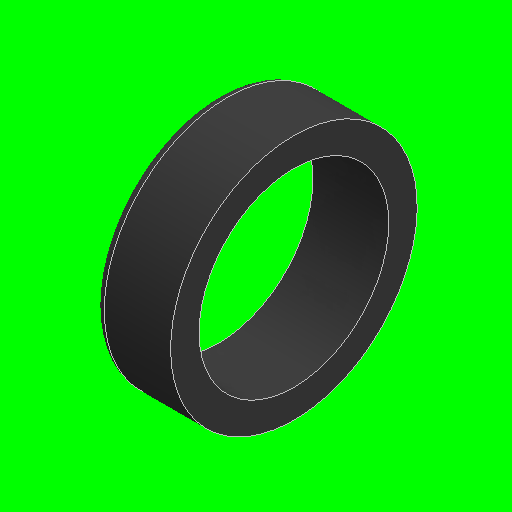
# Autodesk Inventor part: Tire
Saved by Autodesk Inventor 2023 (Build 270158000, 158)
## iProperties
Created: 2022-03-28
Part Number: Tire
Material: ゴム
Document SubType Name: Modeling
Designer: neko2
Density: 0.93 g/cm^3
Appearance: ゴム - 黒
Author: neko2
Autodesk Inventor part; units mm, degrees
ref_plane "YZ Plane" through (0, 0, 0) normal (1, 0, 0) x (0, 1, 0)
ref_plane "XZ Plane" through (0, 0, 0) normal (0, 1, 0) x (-1, 0, 0)
ref_plane "XY Plane" through (0, 0, 0) normal (0, 0, 1) x (1, 0, 0)
sketch "スケッチ1" plane through (0, 0, 0) normal (1, 0, 0) x (0, 1, 0)
  circle A0 centre (0, 0) radius 6.5
  circle A1 centre (0, 0) radius 5
  dimension "d0" = 13
  dimension "d1" = 10
  constraints: 2 centre point, 2 coincident
  measures "d0" diameter of A0
  measures "d1" diameter of A1
extrude "押し出し1" add sketch "スケッチ1" along normal blind 4
fillet "フィレット1" radius 0.5 1 edges at (0, -6.5, 0)
